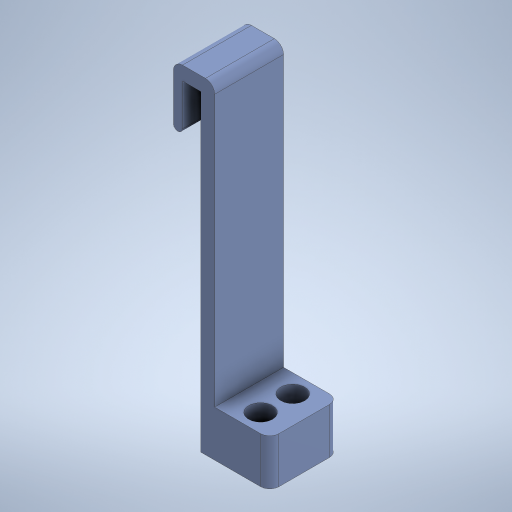
# Autodesk Inventor part: Support_leds_v1
Saved by Autodesk Inventor 2024.1 (Build 281209000, 209)
## iProperties
Created: 2024-05-06
Part Number: Support_leds_v1
Material: Générique
Document SubType Name: Modeling
Designer: chass
Density: 1 g/cm^3
Appearance: Par défaut
Author: chass
## iProperties of the stored document Support_leds_v1_Impression 3D.ipt
Created: 2024-05-13
Part Number: Support_leds_v1_Impression 3D
Material: Générique
Document SubType Name: Modeling
Designer: chass
Density: 1 g/cm^3
Appearance: Par défaut
Author: chass
Autodesk Inventor part; units mm, degrees
ref_plane "YZ Plane" through (0, 0, 0) normal (1, 0, 0) x (0, 1, 0)
ref_plane "XZ Plane" through (0, 0, 0) normal (0, 1, 0) x (-1, 0, 0)
ref_plane "XY Plane" through (0, 0, 0) normal (0, 0, 1) x (1, 0, 0)
sketch "Esquisse1" plane through (0, 0, 0) normal (0, 0, 1) x (1, 0, 0)
  line L0 (-1, 74) -> (-1, 6)
  line L1 (-1, 6) -> (14, 6)
  line L2 (14, 6) -> (14, 16)
  line L3 (14, 16) -> (2, 16)
  line L4 (2, 16) -> (2, 74)
  line L5 (-1, 74) -> (-5, 74)
  line L6 (2, 74) -> (2, 77)
  line L7 (-5, 74) -> (-5, 64)
  line L8 (-5, 64) -> (-7, 64)
  line L9 (-7, 64) -> (-7, 77)
  line L10 (-7, 77) -> (2, 77)
  point P0 (0, 0)
  dimension "d9" = 3
  dimension "d10" = 10
  dimension "d11" = 15
  dimension "d13" = 68
  dimension "d14" = 4
  dimension "d15" = 3
  dimension "d16" = 2
  constraints: 22 end point, 5 perpendicular, 2 horizontal, 2 vertical
  measures "d9" distance of L4.end L0.start
  measures "d10" distance of L1.end L2.end
  measures "d11" distance of L0.end L1.end
  measures "d13" distance of L0.start L0.end
  measures "d14" distance of L0.start L5.end
  measures "d15" distance of L4.end L6.end
  measures "d16" distance of L7.end L8.end
extrude "Extrusion1" add sketch "Esquisse1" along normal blind 15
sketch "Esquisse2" plane through (2, 16, 0) normal (0, 1, 0) x (1, 0, 0)
  circle A0 centre (6, -11) radius 2.6
  circle A1 centre (6, -4) radius 2.6
  line L0 (12, -15) -> (0, -15) projected
  line L1 (12, 0) -> (-2, 0) projected
  line L2 (0, 0) -> (0, -15) projected
  dimension "d2" = 5.2
  dimension "d3" = 5.2
  dimension "d4" = 4
  dimension "d5" = 4
  dimension "d17" = 6
  dimension "d18" = 6
  constraints: 2 centre point
  measures "d2" diameter of A0
  measures "d3" diameter of A1
  measures "d4" distance from line of A0.centre L0
  measures "d5" distance from line of L1 A1.centre
  measures "d17" distance from line of L2 A1.centre
  measures "d18" distance from line of L2 A0.centre
extrude "Extrusion2" cut sketch "Esquisse2" against normal blind 16.25
fillet "Congé2" radius 2 2 edges at (14, 11, 15) (14, 11, 0)
fillet "Congé3" radius 2 2 edges at (-7, 77, 7.5) (2, 77, 7.5)
fillet "Congé4" radius 1 2 edges at (-7, 64, 7.5) (-5, 64, 7.5)
